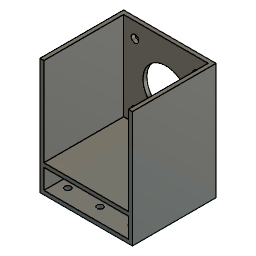
robotic arm assembly (Autodesk Fusion 360 archive; units mm, degrees)
design "bottom motor bracket"
part number: 2026-08-28-15-32-36-786
Autodesk Fusion 360 part; units mm, degrees
sketch "Sketch1" plane through (0, 0, 0) normal (0, 0, 1) x (1, 0, 0)
  line L0 (-21, -23.2) -> (25.4, -23.2)
  line L1 (25.4, 23.2) -> (-21, 23.2)
  line L2 (-14.3858, -20) -> (18.7858, -20)
  line L3 (18.7858, -20) -> (22.2, -16.5858)
  line L4 (-17.8, -16.5858) -> (-14.3858, -20)
  line L5 (25.4, 23.2) -> (27.4, 23.2)
  line L6 (23.4, -21.2) -> (23.4, 21.2)
  line L7 (-21, 23.2) -> (-21, -23.2)
  line L8 (-14.3858, 20) -> (-17.8, 16.5858)
  circle A0 centre (-13.3, -15.5) radius 1.9
  circle A1 centre (-13.3, 15.5) radius 1.9
  line L9 (13.7, 21.2) -> (13.7, 23.2)
  line L10 (-9.3, 0) -> (-9.3, 21.2)
  circle A2 centre (2.2, 0) radius 11
  line L11 (22.2, 16.5858) -> (18.7858, 20)
  line L12 (22.2, -16.5858) -> (22.2, 16.5858)
  line L13 (25.4, -23.2) -> (25.4, 23.2)
  circle A3 centre (17.7, -15.5) radius 1.9
  circle A4 centre (-13.3, 15.5) radius 1.5
  line L14 (-19, -21.2) -> (23.4, -21.2)
  line L15 (-21, -23.2) -> (-21, 23.2)
  line L16 (18.7858, 20) -> (-14.3858, 20)
  circle A5 centre (2.2, 0) radius 11.5
  circle A6 centre (-13.3, -15.5) radius 1.5
  line L17 (13.7, 0) -> (13.7, 21.2)
  line L18 (-19, 21.2) -> (-19, -21.2)
  line L19 (-17.8, 16.5858) -> (-17.8, -16.5858)
  line L20 (23.4, 21.2) -> (-19, 21.2)
  circle A7 centre (17.7, 15.5) radius 1.9
  line L21 (25.4, -23.2) -> (25.4, 23.2)
  line L22 (-9.3, 21.2) -> (-9.3, 23.2)
  line L23 (23.4, 21.2) -> (23.4, 23.2)
  line L24 (27.4, 23.2) -> (27.4, -23.2)
  circle A8 centre (17.7, -15.5) radius 1.5
  line L25 (-19, 21.2) -> (-19, 23.2)
  circle A9 centre (17.7, 15.5) radius 1.5
  line L26 (27.4, -23.2) -> (25.4, -23.2)
  point P0 (-18.8, -21)
  dimension "d1" = 0.5
  dimension "d2" = 0.4
  dimension "d3" = 0.4
  dimension "d4" = 0.4
  dimension "d5" = 0.4
  dimension "d6" = 2
  dimension "d7" = 1.2
  dimension "d8" = 1.2
  dimension "d9" = 1.2
  dimension "d10" = 1.2
  dimension "d11" = 2
  constraint coincident L10.start A5
  constraint coincident L10.end L20
  constraint tangent L10 A5
  constraint coincident L17.start A5
  constraint coincident L9.start L20
  constraint tangent A5 L17
  constraint perpendicular L10 L20
  constraint perpendicular L17 L20
  constraint coincident L22.end L1
  constraint perpendicular L1 L22
  constraint coincident L9.end L1
  constraint perpendicular L1 L9
  constraint coincident L25.end L1
  constraint perpendicular L1 L25
  constraint coincident L23.end L1
  constraint perpendicular L1 L23
  constraint horizontal L5
  constraint vertical L24
  constraint horizontal L26
  constraint vertical L13
  measures "d7" distance of L6 L12
  measures "d8" distance of L16 L20
  measures "d9" distance of L2 L14
  measures "d10" distance of L18 L19
  measures "d11" distance of L5.end L1.start
extrude "Extrude1" add sketch "Sketch1" along normal blind 2 contours L0 L1 L6 L7 L13 L14 L15 L18 L21 L23 L25 | L1 L20 L22 L25 | L1 L9 L20 L23 | L1 L9 L20 L22 | L2 L3 L4 L6 L8 L10 L11 L12 L14 L16 L17 L18 L19 L20 | L10 L16 L17 L20 | L10 L16 A5 L17 | L2 L3 L4 L8 L10 L11 L12 L16 A5 L17 L19 makes body 1
extrude "Extrude2" add sketch "Sketch1" along normal blind 42 contours L0 L1 L6 L7 L13 L14 L15 L18 L21 L23 L25 bodies 1
sketch "Sketch2" plane through (0, -23.2, 0) normal (0, -1, 0) x (1, 0, 0)
  line L0 (-21, 0) -> (25.4, 0)
  line L1 (25.4, 0) -> (25.4, 42)
  line L2 (25.4, 42) -> (-21, 42)
  line L3 (-21, 42) -> (-21, 0)
  circle A0 centre (18.4, 35) radius 1.5
  line L4 (-14, 7) -> (18.4, 7)
  line L5 (18.4, 7) -> (18.4, 35)
  line L6 (18.4, 35) -> (-14, 35)
  line L7 (-14, 35) -> (-14, 7)
  circle A1 centre (2.2, 35) radius 1.5
  circle A2 centre (-14, 35) radius 1.5
  circle A3 centre (18.4, 21) radius 1.5
  circle A4 centre (2.2, 21) radius 1.5
  circle A5 centre (-14, 21) radius 1.5
  circle A6 centre (18.4, 7) radius 1.5
  circle A7 centre (2.2, 7) radius 1.5
  circle A8 centre (-14, 7) radius 1.5
  line L8 (-19, 42) -> (-19, 2)
  line L9 (-19, 2) -> (23.4, 2)
  line L10 (23.4, 2) -> (23.4, 42)
  dimension "d16" = 3
  dimension "d17" = 7
  dimension "d18" = 7
  dimension "d19" = -7
  dimension "d22" = -32.4
  dimension "d23" = -28
  dimension "d27" = -2
  measures "d16" diameter of A0
  measures "d17" distance of L1 A0.centre
  measures "d18" distance of L2 A0.centre
extrude "Extrude3" add sketch "Sketch2" along normal blind 2 from surface at 10 separate body contours L0 L1 L2 L3 L8 L9 L10 | L2 L8 L9 L10 | A0 L4 L5 L6 L7 A1 A2 A3 A5 A6 A7 A8 makes body 2
extrude "Extrude4" add sketch "Sketch2" along normal blind 12 contours L0 L1 L2 L3 L8 L9 L10 bodies 2 1
sketch "Sketch3" plane through (0, -35.2, 0) normal (0, -1, 0) x (1, 0, 0)
  circle A0 centre (2.2, 21) radius 1.5
  circle A1 centre (2.2, 7) radius 1.5
  circle A2 centre (18.4, 35) radius 1.5
  circle A3 centre (-14, 21) radius 1.5
  circle A4 centre (-14, 7) radius 1.5
  circle A5 centre (2.2, 35) radius 1.5
  circle A6 centre (18.4, 7) radius 1.5
  circle A7 centre (-14, 35) radius 1.5
  circle A8 centre (18.4, 21) radius 1.5
  line L0 (25.4, 42) -> (-21, 42)
  line L1 (-21, 42) -> (-21, 0)
  line L2 (-21, 0) -> (25.4, 0)
  line L3 (25.4, 0) -> (25.4, 42)
